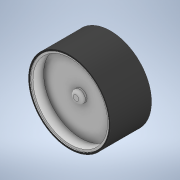
# Autodesk Inventor part: WHEEL 2
Saved by Autodesk Inventor 2022 (Build 260153000, 153)
## iProperties
Created: 2022-08-22
Part Number: WHEEL 2
Material: Generic
Document SubType Name: Modeling
Designer: Sachin
Density: 1 g/cm^3
Appearance: Default
Author: Sachin
Autodesk Inventor part; units mm, degrees
ref_plane "YZ Plane" through (0, 0, 0) normal (1, 0, 0) x (0, 1, 0)
ref_plane "XZ Plane" through (0, 0, 0) normal (0, 1, 0) x (-1, 0, 0)
ref_plane "XY Plane" through (0, 0, 0) normal (0, 0, 1) x (1, 0, 0)
sketch "Sketch1" plane through (0, 0, 0) normal (0, 0, 1) x (1, 0, 0)
  circle A0 centre (0, 0) radius 25
  dimension "d0" = 50
  constraints: 1 centre point, 1 coincident
  measures "d0" diameter of A0
extrude "Extrusion1" add sketch "Sketch1" along normal blind 25
sketch "Sketch2" plane through (0, 0, 25) normal (0, 0, 1) x (1, 0, 0)
  circle A0 centre (0, 0) radius 22.7546
  constraints: 1 centre point, 1 coincident
sketch "Sketch3" plane through (0, 0, 0) normal (0, 0, -1) x (-1, 0, 0)
  circle A0 centre (0, 0) radius 22.7077
  constraints: 1 centre point, 1 coincident
extrude "Extrusion2" cut sketch "Sketch2" against normal blind 7
extrude "Extrusion3" cut sketch "Sketch3" against normal blind 7
sketch "Sketch4" plane through (0, 0, 25) normal (0, 0, 1) x (1, 0, 0)
  circle A0 centre (0, 0) radius 24.0163
  constraints: 1 centre point, 1 coincident
extrude "Extrusion4" cut sketch "Sketch4" against normal blind 0.5
sketch "Sketch5" plane through (0, 0, 18) normal (0, 0, 1) x (1, 0, 0)
  circle A0 centre (0, 0) radius 3
  dimension "d9" = 6
  constraints: 1 centre point, 1 coincident
  measures "d9" diameter of A0
extrude "Extrusion5" cut sketch "Sketch5" against normal blind 25
sketch "Sketch6" plane through (0, 0, 18) normal (0, 0, 1) x (1, 0, 0)
  circle A0 centre (0, 0) radius 3.6832
  constraints: 1 centre point, 1 coincident
extrude "Extrusion6" add sketch "Sketch6" along normal blind 3
fillet "Fillet1" radius 2 1 edges at (-3.6832, 0, 21)
sketch "Sketch7" plane through (0, 0, 18) normal (0, 0, 1) x (1, 0, 0)
  point P0 (0, 0)
sketch "Sketch8" plane through (0, 0, 18) normal (0, 0, 1) x (1, 0, 0)
  point P0 (0, 0)
body "Solid1"
